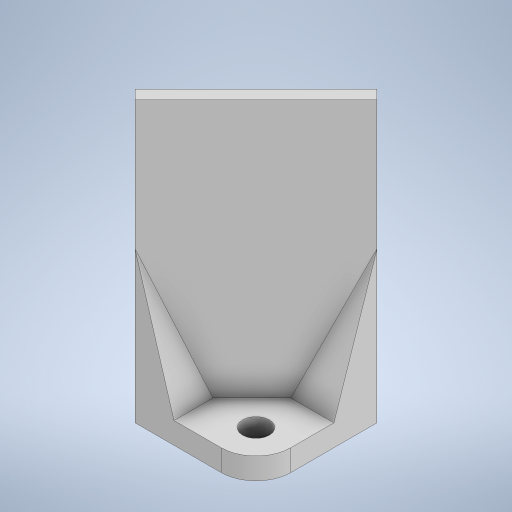
# Autodesk Inventor part: motor_limit_2
Saved by Autodesk Inventor 2024.3 (Build 283343000, 343)
## iProperties
Created: 2025-10-22
Part Number: motor_limit_2
Material: 일반
Document SubType Name: Modeling
Designer: joung
Density: 1 g/cm^3
Appearance: 기본값
Author: joung
Autodesk Inventor part; units mm, degrees
ref_plane "YZ Plane" through (0, 0, 0) normal (1, 0, 0) x (0, 1, 0)
ref_plane "XZ Plane" through (0, 0, 0) normal (0, 1, 0) x (-1, 0, 0)
ref_plane "XY Plane" through (0, 0, 0) normal (0, 0, 1) x (1, 0, 0)
sketch "스케치1" plane through (0, 0, 0) normal (0, 1, 0) x (-1, 0, 0)
  circle A0 centre (0, 0) radius 3.1
  circle A1 centre (0, 0) radius 8.1
  line L0 (-8.1, 0) -> (-8.1, -20)
  line L1 (0, 8.1) -> (20, 8.1)
  line L2 (20, 8.1) -> (-8.1, -20)
  line L3 (20, 8.1) -> (22.1213, 5.9787)
  line L4 (22.1213, 5.9787) -> (-5.9787, -22.1213)
  line L5 (-5.9787, -22.1213) -> (-8.1, -20)
  dimension "d0" = 6.2
  dimension "d1" = 5
  dimension "d2" = 20
  dimension "d3" = 20
  dimension "d4" = 3
  constraints: 12 end point, 3 perpendicular, 2 centre point, 2 point on circle, 1 coincident, 1 horizontal, 1 tangent, 1 vertical
  measures "d0" diameter of A0
  measures "d1" radial gap between concentric circles of A0 A1
  measures "d2" distance of L0.start L0.end
  measures "d3" distance of L1.start L1.end
  measures "d4" distance of L1.end L3.end
extrude "돌출1" add sketch "스케치1" along normal blind 5
sketch "스케치2" plane through (0, 5, 0) normal (0, 1, 0) x (1, 0, 0)
  line L0 (-22.1213, -5.9787) -> (-20, -8.1) projected
  line L1 (-20, -8.1) -> (8.1, 20)
  line L2 (5.9787, 22.1213) -> (-22.1213, -5.9787) projected
  line L3 (8.1, 20) -> (5.9787, 22.1213)
  line L4 (5.9787, 22.1213) -> (-22.1213, -5.9787)
  line L5 (-22.1213, -5.9787) -> (-20, -8.1)
  point P0 (0, 0)
  constraints: 8 end point, 2 equal length, 2 perpendicular
extrude "돌출2" add sketch "스케치2" along normal blind 60
sketch "스케치3" plane through (8.1, 0, 0) normal (1, 0, 0) x (0, 0, -1)
  line L0 (0, 5) -> (20, 5) projected
  line L1 (10, 5) -> (20, 35)
  line L2 (20, 5) -> (20, 65) projected
  line L3 (10, 5) -> (20, 5)
  line L4 (20, 5) -> (20, 35)
  point P0 (0, 0)
  constraints: 6 end point, 2 midpoint, 1 horizontal, 1 perpendicular
extrude "돌출3" add sketch "스케치3" against normal blind 10
sketch "스케치4" plane through (-20, 0, 8.1) normal (0, 0, 1) x (1, 0, 0)
  line L0 (18.1, 5) -> (0, 5) projected
  line L1 (9.05, 5) -> (0, 35)
  line L2 (0, 5) -> (0, 65) projected
  line L3 (9.05, 5) -> (0, 5)
  line L4 (0, 5) -> (0, 35)
  point P0 (20, 0)
  constraints: 6 end point, 2 midpoint, 1 horizontal, 1 perpendicular
extrude "돌출4" add sketch "스케치4" against normal blind 10
sketch "스케치5" plane through (-22.1213, 0, 5.9787) normal (-0.7071, 0, 0.7071) x (0.7071, 0, 0.7071)
  line L0 (3, 0) -> (0, 0) projected
  line L1 (0, 35) -> (-4.0711, 35) projected
  line L2 (0, 0) -> (-4.0711, 0)
  line L3 (-4.0711, 0) -> (-4.0711, 35)
  line L4 (-4.0711, 35) -> (0, 35)
  line L5 (0, 35) -> (0, 0)
  point P0 (11.4146, 0)
  constraints: 8 end point, 2 parallel, 1 horizontal, 1 perpendicular
extrude "돌출5" cut sketch "스케치5" against normal through all
